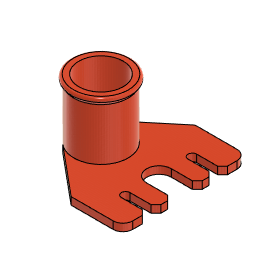
Loom Buddy II v4 (Autodesk Fusion 360 design; units mm, degrees)
Autodesk Fusion 360 part; units mm, degrees
ref_plane "WorkPlane1" through (-5.5, -13.5, 34.515) normal (0, 0, 1) x (1, 0, 0)
sketch "Lost plane" plane through (-5.5, 14.3492, 34.515) normal (0, 0, 1) x (1, 0, 0)
  line L0 (10.5, 10.7658) -> (-18.5, 10.7658)
  line L1 (-18.5, 10.7658) -> (-18.5, -39.4642) construction
  line L2 (-18.5, -39.4642) -> (10.5, -39.4642)
  line L3 (10.5, -39.4642) -> (10.5, 10.7658)
  circle A0 centre (0, -0.8492) radius 1.75
  circle A1 centre (0, -27.8492) radius 1.75
  line L4 (10.5, -14.3492) -> (-18.5, -14.3492) construction
  circle A2 centre (0, -27.8492) radius 3.5 construction
  line L5 (16.5, 5.6508) -> (18.5, 7.6508)
  circle A3 centre (24.4, -4.3492) radius 1.25
  circle A4 centre (24.4, -24.3492) radius 1.25
  line L6 (10.5, -28.3492) -> (16.5, -34.3492)
  line L7 (16.5, 5.6508) -> (10.5, -0.3492)
  line L8 (18.5, -36.3492) -> (16.5, -34.3492)
  line L9 (-18.5, -21.3492) -> (-18.5, -7.3492)
  line L10 (-18.5, -24.3492) -> (-18.5, -21.3492)
  line L11 (-18.5, -7.3492) -> (-18.5, -4.3492)
  line L12 (-18.5, -4.3492) -> (-14.5, -0.3492)
  line L13 (-10.5, -0.3492) -> (-14.5, -0.3492)
  line L14 (-10.5, -0.3492) -> (-10.5, 12.7658)
  line L15 (-5.7, 12.7658) -> (-5.7, 10.7658)
  line L16 (5.7, 10.7658) -> (5.7, 12.7658)
  line L17 (10.5, -0.3492) -> (10.5, 12.7658)
  line L18 (-14.5, -28.3492) -> (-18.5, -24.3492)
  line L19 (-10.5, -28.3492) -> (-14.5, -28.3492)
  line L20 (10.5, -41.4642) -> (10.5, -28.3492)
  line L21 (5.7, -41.4642) -> (5.7, -39.4642)
  line L22 (-5.7, -39.4642) -> (-5.7, -41.4642)
  line L23 (-10.5, -41.4642) -> (-10.5, -28.3492)
  line L24 (-5.7, -39.4642) -> (5.7, -39.4642)
  line L25 (-10.5, -43.4642) -> (-10.5, -41.4642)
  line L26 (10.5, 14.7658) -> (10.5, 12.7658)
  line L27 (-10.5, 12.7658) -> (-10.5, 14.7658)
  line L28 (-5.7, -41.4642) -> (-5.7, -43.4642)
  line L29 (-5.7, -43.4642) -> (-10.5, -43.4642)
  line L30 (10.5, -43.4642) -> (5.7, -43.4642)
  line L31 (5.7, -43.4642) -> (5.7, -41.4642)
  line L32 (5.7, 12.7658) -> (5.7, 14.7658)
  line L33 (5.7, 14.7658) -> (10.5, 14.7658)
  line L34 (-10.5, 14.7658) -> (-5.7, 14.7658)
  line L35 (-5.7, 14.7658) -> (-5.7, 12.7658)
  line L36 (10.5, -41.4642) -> (10.5, -43.4642)
  circle A5 centre (0, -27.8492) radius 1.5 construction
  circle A6 centre (0, -0.8492) radius 1.5 construction
  line L37 (-5.7, 10.7658) -> (5.7, 10.7658)
  line L38 (0, -0.8492) -> (0, -27.8492) construction
  circle A7 centre (0, -14.3492) radius 5
  line L39 (0, -9.3492) -> (10.5, -9.3492)
  line L40 (0, -19.3492) -> (10.5, -19.3492)
  line L41 (0, 0.9008) -> (10.5, 0.9008)
  line L42 (0, -2.5992) -> (10.5, -2.5992)
  line L43 (0, -26.0992) -> (10.5, -26.0992)
  line L44 (0, -29.5992) -> (10.5, -29.5992)
  line L45 (-10.5, -0.3492) -> (-10.5, -28.3492)
  dimension "d5291" = 29
  dimension "d5294" = 3.5
  dimension "d5295" = 3.5
  dimension "d5311" = 7
  dimension "d7129" = 10
  dimension "d7130" = 6.75
  constraint horizontal L0
  constraint vertical L1
  constraint horizontal L2
  constraint vertical L3
  constraint midpoint L3 L4.start
  constraint midpoint L4.end L9
  constraint concentric A1 A2
  constraint coincident A1.centre A2.centre
  constraint coincident A0.centre A6.centre
  constraint horizontal L4
  constraint coincident L0.start L17
  constraint coincident L0 L15.end
  constraint midpoint L38 A7.centre
  constraint coincident A7 L39.start
  constraint tangent A7 L39
  constraint coincident L3 L39.end
  constraint perpendicular L3 L39
  constraint coincident A7 L40.start
  constraint tangent A7 L40
  constraint coincident L3 L40.end
  constraint perpendicular L3 L40
  constraint coincident A0 L41.start
  constraint tangent A0 L41
  constraint perpendicular L17 L41
  constraint coincident A0 L42.start
  constraint tangent A0 L42
  constraint coincident L3 L42.end
  constraint perpendicular L3 L42
  constraint coincident L3 L41.end
  constraint coincident A1 L43.start
  constraint coincident L38 L43.start
  constraint coincident L3 L43.end
  constraint tangent A1 L43
  constraint coincident A1 L44.start
  constraint tangent A1 L44
  constraint perpendicular L20 L44
  constraint coincident L3 L44.end
  constraint coincident L13.start L14.start
  constraint coincident L19.start L23.end
  measures "d5291" distance of L1.end L2.end
  measures "d5294" diameter of A0
  measures "d5295" diameter of A1
  measures "d5311" diameter of A2
  measures "d7129" diameter of A7
  measures "d7130" distance of L39 L42
extrude "Extrude1" add sketch "Lost plane" along normal blind 3 contours L0 L2 L3 A0 A1 L14 L17 L20 L23 L24 L37 A7 L39 L40 L41 L42 L43 L44 L45
fillet "Fillet7" radius 4 2 edges at (5, -25.115, 36.015) (5, 25.115, 36.015)
sketch "Sketch19" plane through (0, 0, 37.515) normal (0, 0, 1) x (-1, 0, 0)
  line L0 (16, 25.115) -> (-1, 25.115)
  line L1 (-5, 21.115) -> (-5, 15.25)
  line L2 (-1, -25.115) -> (-0.2, -25.115)
  line L3 (0, 0) -> (29, 0) construction
  circle A0 centre (29, 0) radius 11
  circle A1 centre (29, 0) radius 9
  line L4 (36.0328, -8.4581) -> (16, -25.115)
  arc A2 (-5, -21.115) -> (-1, -25.115) centre (-1, -21.115) ccw
  arc A3 (-1, 25.115) -> (-5, 21.115) centre (-1, 21.115) ccw
  line L5 (16, -25.115) -> (16, 25.115)
  line L6 (-0.2, -25.115) -> (11.2, -25.115)
  line L7 (11.2, -25.115) -> (16, -25.115)
  line L8 (-5, 15.25) -> (5.5, 15.25)
  arc A4 (5.5, 11.75) -> (5.5, 15.25) centre (5.5, 13.5) ccw
  line L9 (5.5, 11.75) -> (-5, 11.75)
  line L10 (-5, 11.75) -> (-5, 5)
  line L11 (-5, 5) -> (5.5, 5)
  arc A5 (5.5, -5) -> (5.5, 5) centre (5.5, 0) ccw
  line L12 (5.5, -5) -> (-5, -5)
  line L13 (-5, -5) -> (-5, -11.75)
  line L14 (-5, -11.75) -> (5.5, -11.75)
  arc A6 (5.5, -15.25) -> (5.5, -11.75) centre (5.5, -13.5) ccw
  line L15 (5.5, -15.25) -> (-5, -15.25)
  line L16 (-5, -15.25) -> (-5, -21.115)
  line L17 (36.0328, 8.4581) -> (16, 25.115)
  dimension "d6638" = 2
  dimension "d6639" = 18
  dimension "d6740" = 22
  dimension "d7127" = 2
  constraint horizontal L3
  constraint coincident L3.end A0.centre
  constraint concentric A0 A1
  constraint coincident A0 L4.start
  constraint tangent A0 L4
  constraint coincident L4.end L5.start
  constraint coincident L3.start origin
  constraint coincident A0 L17.start
  constraint tangent A0 L17
  constraint coincident L0.start L5.end
  measures "d6638" distance of A0 A1
  measures "d6639" diameter of A1
  measures "d6740" diameter of A0
  measures "d7127" distance of A0 L5
extrude "Extrude21" add sketch "Sketch19" against normal blind 3 contours A0 L4 L5 L17 | A0
extrude "Extrude22" add sketch "Sketch19" along normal blind 24 contours A0
ref_plane "WorkPlane7" through (-29, 0, 71.015) normal (0, 1, 0) x (0, 0, -1)
sketch "Sketch22" plane through (-26, 0, 69.015) normal (0, 1, 0) x (1, 0, 0)
  line L0 (-14, 7.5) -> (8, 7.5)
  line L1 (-10.0328, 31.5) -> (-10.0328, 34.5)
  line L2 (-10.0328, 34.5) -> (-14, 34.5)
  line L3 (8, 31.5) -> (-10.0328, 31.5)
  line L4 (-14, 7.5) -> (-16, 7.5)
  line L5 (-16, 7.5) -> (-14, 10.5)
  line L6 (-14, 7.5) -> (8, 7.5)
  line L7 (-10.0328, 34.5) -> (-14, 34.5)
  line L8 (8, 7.5) -> (8, 31.5)
  line L9 (-14, 7.5) -> (-14, 34.5)
  line L10 (-10.0328, 34.5) -> (-10.0328, 31.5)
  line L11 (8, 31.5) -> (10, 31.5)
  line L12 (10, 34.5) -> (-10.0328, 34.5)
  line L13 (10, 31.5) -> (27, 31.5)
  line L14 (31, 31.5) -> (27, 31.5)
  line L15 (27, 34.5) -> (31, 34.5)
  line L16 (10, 34.5) -> (27, 34.5)
  line L17 (31, 34.5) -> (31, 31.5)
  dimension "d6743" = 2
  dimension "d6744" = 33.7
  dimension "d6745" = 3
  constraint coincident L0.start L4.start
  constraint parallel L0 L4
  constraint coincident L5.end L9
  measures "d6743" distance of L0.start L4.end
  measures "d6745" distance of L0.start L5.end
revolve "Revolve2" add sketch "Sketch22" angle 360 about axis through (-29, 0, 37.515) along (0, 0, -1) contours L4 L5 L9
fillet "Fillet8" radius 1 1 edges at (-41.1203, 4.701, 61.515)
chamfer "Chamfer17" distance 2 angle 45 6 edges at (5, -11.75, 36.015) (5, -15.25, 36.015) (5, 5, 36.015) (5, -5, 36.015) (5, 11.75, 36.015) (5, 15.25, 36.015)
named bodies: "Loom Buddy_1x_SN"
